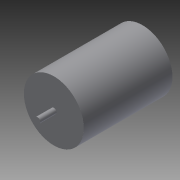
# Autodesk Inventor part: Motor
Saved by Autodesk Inventor 2015 SP1 (Build 190203100, 203)
## iProperties
Created: 2016-02-02
Part Number: Motor
Material: Generic
Document SubType Name: Modeling
Designer: tuttlem
Density: 1 g/cm^3
Appearance: Default
Author: tuttlem
Autodesk Inventor part; units mm, degrees
ref_plane "YZ Plane" through (0, 0, 0) normal (1, 0, 0) x (0, 1, 0)
ref_plane "XZ Plane" through (0, 0, 0) normal (0, 1, 0) x (-1, 0, 0)
ref_plane "XY Plane" through (0, 0, 0) normal (0, 0, 1) x (1, 0, 0)
sketch "Sketch1" plane through (0, 0, 0) normal (0, 1, 0) x (-1, 0, 0)
  line L0 (240.1229, 0) -> (152.4929, 0)
  line L1 (152.4929, 0) -> (152.4929, -259.08)
  line L2 (152.4929, -259.08) -> (240.1229, -259.08)
  line L3 (240.1229, -259.08) -> (240.1229, 0)
  point P0 (0, 0)
  dimension "d0" = 259.08
  dimension "d1" = 87.63
  constraints: 8 end point, 2 parallel, 1 horizontal, 1 perpendicular
  measures "d0" distance of L2.end L0.start
  measures "d1" distance of L1.end L2.end
revolve "Revolution1" add sketch "Sketch1" angle 360 about axis through (-152.4929, 0, 0) along (0, 0, -1)
sketch "Sketch2" plane through (-152.4929, 0, 0) normal (0, 0, 1) x (1, 0, 0)
  circle A0 centre (0, 0) radius 7.9375
  point P0 (152.4929, 0)
  dimension "d3" = 15.875
  constraints: 1 centre point
  measures "d3" diameter of A0
extrude "Extrusion1" add sketch "Sketch2" along normal blind 47.752
body "Solid1"
